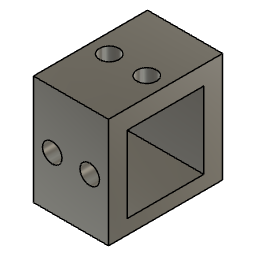
모터브라켓-B (Autodesk Fusion 360 design; units mm, degrees)
Autodesk Fusion 360 part; units mm, degrees
sketch "스케치1" plane through (0, 0, 0) normal (1, 0, 0) x (0, 1, 0)
  line L0 (15.2, 15.2) -> (-15.2, 15.2)
  line L1 (-15.2, 15.2) -> (-15.2, -15.2)
  line L2 (-15.2, -15.2) -> (15.2, -15.2)
  line L3 (15.2, -15.2) -> (15.2, 15.2)
  line L4 (15.2, 15.2) -> (-15.2, -15.2) construction
  line L5 (-15.2, 15.2) -> (15.2, -15.2) construction
  line L6 (10.2, 10.2) -> (-10.2, 10.2)
  line L7 (-10.2, 10.2) -> (-10.2, -10.2)
  line L8 (-10.2, -10.2) -> (10.2, -10.2)
  line L9 (10.2, -10.2) -> (10.2, 10.2)
  line L10 (10.2, 10.2) -> (-10.2, -10.2) construction
  line L11 (-10.2, 10.2) -> (10.2, -10.2) construction
  dimension "d1" = 30.4
  dimension "d2" = 30.4
  dimension "d3" = 20.4
  dimension "d4" = 20.4
  constraint horizontal L0
  constraint perpendicular L0 L1
  constraint parallel L0 L2
  constraint parallel L1 L3
  constraint coincident L4 origin
  constraint coincident L5 origin
  constraint horizontal L6
  constraint perpendicular L6 L7
  constraint parallel L6 L8
  constraint parallel L7 L9
  constraint coincident L10 origin
  constraint coincident L11 origin
  measures "d1" distance of L1.end L2.end
  measures "d2" distance of L0.end L1.end
  measures "d3" distance of L7.end L8.end
  measures "d4" distance of L6.end L7.end
extrude "돌출1" add sketch "스케치1" along normal blind 20
extrude "돌출2" cut 1 faces at (13.3333, -5.0667, -15.2) along direction (0, 0, 1) blind 1.2
sketch "스케치2" plane through (0, 0, 15.2) normal (0, 0, 1) x (-1, 0, 0)
  line L0 (0, -15.2) -> (0, 15.2)
  line L1 (0, 15.2) -> (-20, 15.2)
  line L2 (-20, 15.2) -> (-20, -15.2)
  line L3 (-20, -15.2) -> (0, -15.2)
  line L4 (0, 0) -> (-5, 0)
  circle A0 centre (-5, 0) radius 2.6
  line L5 (-20, 0) -> (-15, 0)
  circle A1 centre (-15, 0) radius 2.6
  dimension "d9" = 5
  dimension "d10" = 5.2
  dimension "d11" = 5
  dimension "d12" = 5.2
  constraint coincident L4.start origin
  constraint perpendicular L0 L4
  constraint coincident L4.end A0.centre
  constraint midpoint L2 L5.start
  constraint perpendicular L2 L5
  constraint coincident L5.end A1.centre
  measures "d9" distance of L4.start L4.end
  measures "d10" diameter of A0
  measures "d11" distance of L5.start L5.end
  measures "d12" diameter of A1
extrude "돌출3" cut sketch "스케치2" against normal blind 10 contours A0 | A1
sketch "스케치3" plane through (0, -15.2, 0) normal (0, -1, 0) x (1, 0, 0)
  line L0 (0, -14) -> (20, -14)
  line L1 (20, -14) -> (20, 15.2)
  line L2 (20, 15.2) -> (0, 15.2)
  line L3 (0, 15.2) -> (0, -14)
  line L4 (0, 0) -> (5, 0)
  line L5 (20, 0) -> (15, 0)
  circle A0 centre (5, 0) radius 2.6
  circle A1 centre (15, 0) radius 2.6
  dimension "d15" = 5
  dimension "d16" = 5
  dimension "d17" = 5.2
  dimension "d18" = 5.2
  constraint coincident L4.start origin
  constraint horizontal L4
  constraint coincident L1 L5.start
  constraint perpendicular L1 L5
  constraint coincident L4.end A0.centre
  constraint coincident L5.end A1.centre
  measures "d15" distance of L4.start L4.end
  measures "d16" distance of L5.start L5.end
  measures "d17" diameter of A0
  measures "d18" diameter of A1
extrude "돌출4" cut sketch "스케치3" against normal blind 5 contours A0 | A1
